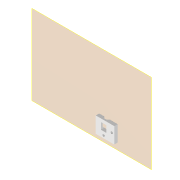
# Autodesk Inventor part: 20_Scanner_Fixation
Saved by Autodesk Inventor 2022 (Build 260153000, 153)
## iProperties
Created: 2022-09-19
Part Number: 20_Scanner_Fixation
Material: Generisch
Document SubType Name: Modeling
Designer: UC2
Density: 1 g/cm^3
Appearance: Vorgabe
Author: UC2
Autodesk Inventor part; units mm, degrees
ref_plane "YZ Plane" through (0, 0, 0) normal (1, 0, 0) x (0, 1, 0)
ref_plane "XZ Plane" through (0, 0, 0) normal (0, 1, 0) x (-1, 0, 0)
ref_plane "XY Plane" through (0, 0, 0) normal (0, 0, 1) x (1, 0, 0)
ref_plane "Arbeitsebene1" through (0, 0, 0) normal (0, 0, 1) x (1, 0, 0)
sketch "Skizze1" plane through (0, 0, 0) normal (0, 0, 1) x (1, 0, 0)
  circle A0 centre (5.4922, -12.0867) radius 1.4 projected
  circle A1 centre (17.95, -36.25) radius 1.4 projected
  circle A2 centre (-27.8589, -14.9953) radius 1.4 projected
  circle A3 centre (-42.2276, -36.25) radius 1.4 projected
  circle A4 centre (-42.2276, -19.25) radius 1.4 projected
  circle A5 centre (-27.8589, -39.949) radius 1.4 projected
  circle A6 centre (27.4914, -28.65) radius 1.4 projected
  circle A7 centre (32.285, -12.0867) radius 1.4 projected
  line L0 (-8.36, -23.75) -> (8.8222, -23.75) projected
  line L1 (8.8222, -23.75) -> (8.8222, -7.25) projected
  line L2 (8.8222, -7.25) -> (-9.1, -7.25) projected
  line L3 (-9.1, -7.25) -> (-9.1, 29.75) projected
  line L4 (-9.1, 29.75) -> (45.9, 29.75) projected
  line L5 (45.9, 29.75) -> (45.9, -7.25) projected
  line L6 (45.9, -7.25) -> (27.9778, -7.25) projected
  line L7 (27.9778, -7.25) -> (27.9778, -25.25) projected
  line L8 (27.9778, -25.25) -> (21.15, -25.25) projected
  line L9 (21.15, -25.25) -> (21.15, -32.05) projected
  line L10 (21.15, -32.05) -> (14.75, -32.05) projected
  line L11 (14.75, -32.05) -> (14.75, -31.75) projected
  line L12 (14.75, -31.75) -> (-8.36, -31.75) projected
  line L13 (-8.36, -31.75) -> (-8.36, -36.25) projected
  line L14 (-8.36, -36.25) -> (-23.36, -36.25) projected
  line L15 (-23.36, -33.75) -> (-23.36, -36.25) projected
  line L16 (-38.36, -33.75) -> (-23.36, -33.75) projected
  line L17 (-38.36, -33.75) -> (-38.36, -31.25) projected
  line L18 (-38.36, -31.25) -> (-41.36, -31.25) projected
  line L19 (-41.36, -31.25) -> (-41.36, -32.5058) projected
  line L20 (-41.36, -32.5058) -> (-63.9, -32.5058) projected
  line L21 (-63.9, -32.5058) -> (-63.9, -38.75) projected
  arc A8 (-63.9, -38.75) -> (-59.9, -42.75) centre (-59.9, -38.75) ccw projected
  line L22 (-59.9, -42.75) -> (59.9, -42.75) projected
  arc A9 (59.9, -42.75) -> (63.9, -38.75) centre (59.9, -38.75) ccw projected
  line L23 (63.9, -38.75) -> (63.9, 3.9837) projected
  line L24 (63.9, 3.9837) -> (56.9, 3.9837) projected
  line L25 (56.9, 3.9837) -> (56.9, 8.0046) projected
  spline S0 degree 2 poles (56.9, 8.0046) (47.4544, 9.25) (56.9, 10.4954) knots 0.408689 0.408689 0.408689 2.009633 2.009633 2.009633 weights 1.06106 1.156332 1.06106 projected
  line L26 (56.9, 10.4954) -> (56.9, 14.5163) projected
  line L27 (56.9, 14.5163) -> (63.9, 14.5163) projected
  line L28 (63.9, 14.5163) -> (63.9, 38.75) projected
  arc A10 (63.9, 38.75) -> (59.9, 42.75) centre (59.9, 38.75) ccw projected
  line L29 (59.9, 42.75) -> (-59.9, 42.75) projected
  arc A11 (-59.9, 42.75) -> (-63.9, 38.75) centre (-59.9, 38.75) ccw projected
  line L30 (-63.9, 38.75) -> (-63.9, 25.4963) projected
  line L31 (-63.9, 25.4963) -> (-55.9, 25.4963) projected
  line L32 (-55.9, 25.4963) -> (-55.9, 19.75) projected
  line L33 (-55.9, 19.75) -> (-18.9, 19.75) projected
  line L34 (-18.9, 19.75) -> (-18.9, 10.3274) projected
  spline S1 degree 2 poles (-18.9, 10.3274) (-11.6855, 9.25) (-18.9, 8.1726) knots 0.06387 0.06387 0.06387 0.952272 0.952272 0.952272 weights 1.010578 1.079212 1.010578 projected
  line L35 (-18.9, 8.1726) -> (-18.9, -1.25) projected
  line L36 (-18.9, -1.25) -> (-55.9, -1.25) projected
  line L37 (-55.9, -1.25) -> (-55.9, -6.9963) projected
  line L38 (-55.9, -6.9963) -> (-63.9, -6.9963) projected
  line L39 (-63.9, -6.9963) -> (-63.9, -22.9942) projected
  line L40 (-63.9, -22.9942) -> (-41.36, -22.9942) projected
  line L41 (-41.36, -22.9942) -> (-41.36, -24.25) projected
  line L42 (-41.36, -24.25) -> (-38.36, -24.25) projected
  line L43 (-38.36, -24.25) -> (-38.36, -21.75) projected
  line L44 (-38.36, -21.75) -> (-23.36, -21.75) projected
  line L45 (-23.36, -19.25) -> (-23.36, -21.75) projected
  line L46 (-23.36, -19.25) -> (-8.36, -19.25) projected
  line L47 (-8.36, -19.25) -> (-8.36, -23.75) projected
  line L48 (14.75, -32.05) -> (21.15, -32.05)
  line L49 (21.15, -32.05) -> (21.15, -24.25)
  line L50 (21.15, -24.25) -> (14.75, -24.25)
  line L51 (14.75, -24.25) -> (14.75, -32.05)
  line L52 (8.8222, -20.5) -> (30.4914, -20.5)
  line L53 (30.4914, -20.5) -> (30.4914, -39.25)
  line L54 (30.4914, -39.25) -> (8.8222, -39.25)
  line L55 (8.8222, -39.25) -> (8.8222, -20.5)
  point P0 (0, 0)
  point P1 (15.25, -24.75)
  dimension "d0" = 0.5
  dimension "d1" = 3
  dimension "d2" = 3
  constraints: 16 end point, 4 parallel, 2 horizontal, 2 perpendicular, 1 point on line, 1 other
  measures "d0" distance from line of L50 point (15.25, -24.75)
  measures "d1" distance from line of L53 A6.centre
  measures "d2" distance from line of L54 A1.centre
extrude "Extrusion1" add sketch "Skizze1" along normal blind 4 contours L1 L52 L7 L8 L49 L50 L51 L12 L55 | L12 L11 L10 L9 L8 L7 L52 L53 L54 L55
sketch "Skizze2" plane through (0, 0, 0) normal (0, 0, -1) x (-1, 0, 0)
  line L0 (-8.8222, -39.25) -> (-30.4914, -39.25) projected
  line L1 (-8.8222, -20.5) -> (-8.8222, -39.25) projected
  line L2 (-30.4914, -20.5) -> (-8.8222, -20.5) projected
  line L3 (-30.4914, -39.25) -> (-30.4914, -20.5) projected
  line L4 (-14.75, -32.05) -> (-14.75, -24.25) projected
  line L5 (-21.15, -32.05) -> (-14.75, -32.05) projected
  line L6 (-21.15, -24.25) -> (-21.15, -32.05) projected
  line L7 (-14.75, -24.25) -> (-21.15, -24.25) projected
  circle A0 centre (-27.4914, -28.65) radius 1.4 projected
  circle A1 centre (-17.95, -36.25) radius 1.4 projected
  line L8 (-14.75, -32.05) -> (-14.75, -24.25) projected
  line L9 (-8.8222, -20.5) -> (-8.8222, -39.25) projected
  line L10 (-14.75, -27.25) -> (-8.8222, -27.25)
  line L11 (-8.8222, -27.25) -> (-8.8222, -30.05)
  line L12 (-8.8222, -30.05) -> (-14.75, -30.05)
  line L13 (-14.75, -30.05) -> (-14.75, -27.25)
  line L14 (-14.75, -24.25) -> (-21.15, -24.25) projected
  line L15 (-30.4914, -20.5) -> (-8.8222, -20.5) projected
  line L16 (-19.35, -24.25) -> (-16.55, -24.25)
  line L17 (-16.55, -24.25) -> (-16.55, -20.5)
  line L18 (-16.55, -20.5) -> (-19.35, -20.5)
  line L19 (-19.35, -20.5) -> (-19.35, -24.25)
  point P0 (0, 0)
  constraints: 16 end point, 4 parallel, 4 point on line, 2 horizontal, 2 perpendicular
extrude "Extrusion2" cut sketch "Skizze2" against normal blind 2 contours L12 L4 L10 L1 | L2 L17 L7 L19
chamfer "Fase1" distance 1.8 angle 45 4 edges at (11.7861, -30.05, 0) (11.7861, -27.25, 0) (16.55, -22.375, 0) (19.35, -22.375, 0)
